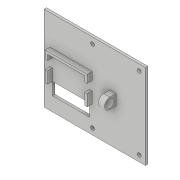
# Autodesk Inventor part: middleBase
Saved by Autodesk Inventor 2019 (Build 230136000, 136)
## iProperties
Created: 2021-03-03
Part Number: middleBase
Material: Generic
Document SubType Name: Modeling
Designer: LuoYi
Density: 1 g/cm^3
Appearance: Default
Author: LuoYi
Autodesk Inventor part; units mm, degrees
ref_plane "YZ Plane" through (0, 0, 0) normal (1, 0, 0) x (0, 1, 0)
sketch "Sketch1" plane through (0, 0, 0) normal (0, 0, 1) x (1, 0, 0)
  line L0 (0, 0) -> (83.5, 0)
  line L1 (83.5, 0) -> (83.5, 70)
  line L2 (83.5, 70) -> (0, 70)
  line L3 (0, 70) -> (0, 0)
  dimension "d0" = 70
  dimension "d1" = 83.5
  constraints: 8 end point, 2 parallel, 1 horizontal, 1 perpendicular
  measures "d0" distance of L2.end L0.start
  measures "d1" distance of L0.start L0.end
extrude "Extrusion1" add sketch "Sketch1" along normal blind 2
sketch "Sketch2" plane through (0, 0, 2) normal (0, 0, 1) x (1, 0, 0)
  line L0 (0, 70) -> (0, 0) projected
  line L1 (0, 35) -> (83.5, 35) construction
  line L2 (83.5, 0) -> (83.5, 70) projected
  line L3 (6.95, 31.4) -> (-5, 31.4) construction
  line L4 (-5, 31.4) -> (-5, 38.6) construction
  line L5 (-5, 38.6) -> (6.95, 38.6) construction
  line L6 (6.95, 38.6) -> (6.95, 31.4) construction
  line L7 (6.95, 31.4) -> (-5, 38.6) construction
  line L8 (-5, 31.4) -> (6.95, 38.6) construction
  line L9 (49.5, 34.65) -> (49.5, 29.45) construction
  line L10 (6.95, 31.4) -> (4.95, 31.4)
  line L11 (4.95, 31.4) -> (4.95, 21.85)
  line L12 (4.95, 21.85) -> (6.95, 21.85)
  line L13 (6.95, 21.85) -> (6.95, 31.4)
  line L14 (6.95, 38.6) -> (4.95, 38.6)
  line L15 (4.95, 38.6) -> (4.95, 45.2)
  line L16 (4.95, 45.2) -> (6.95, 45.2)
  line L17 (6.95, 45.2) -> (6.95, 38.6)
  line L18 (6.95, 45.2) -> (37.55, 45.2)
  line L19 (37.55, 45.2) -> (37.55, 43.2)
  line L20 (37.55, 43.2) -> (6.95, 43.2)
  line L21 (6.95, 43.2) -> (6.95, 45.2)
  line L22 (37.55, 45.2) -> (39.55, 45.2)
  line L23 (39.55, 45.2) -> (39.55, 38.6)
  line L24 (39.55, 38.6) -> (37.55, 38.6)
  line L25 (37.55, 38.6) -> (37.55, 45.2)
  line L26 (37.55, 31.4) -> (39.55, 31.4)
  line L27 (39.55, 31.4) -> (39.55, 21.85)
  line L28 (39.55, 21.85) -> (37.55, 21.85)
  line L29 (37.55, 21.85) -> (37.55, 31.4)
  line L30 (6.95, 21.85) -> (37.55, 21.85)
  line L31 (37.55, 21.85) -> (37.55, 11.6)
  line L32 (37.55, 11.6) -> (6.95, 11.6)
  line L33 (6.95, 11.6) -> (6.95, 21.85)
  point P0 (0.975, 35)
  dimension "d8" = 7.2
  dimension "d13" = 11.95
  dimension "d14" = 5
  dimension "d19" = 2
  dimension "d20" = 23.4
  dimension "d21" = 10.25
  dimension "d22" = 30.6
  dimension "d23" = 2
  dimension "d24" = 2
  dimension "d25" = 33.6
  dimension "d30" = 11.95
  constraints: 64 end point, 14 parallel, 8 point on line, 7 horizontal, 7 perpendicular, 4 midpoint
  measures "d8" distance between parallel lines of L3 L5
  measures "d13" distance between parallel lines of L6 L4
  measures "d14" distance between parallel lines of L0 L4
  measures "d19" distance between parallel lines of L15 L17
  measures "d20" distance between parallel lines of L32 L1
  measures "d21" distance between parallel lines of L32 L30
  measures "d22" distance between parallel lines of L25 L17
  measures "d23" distance between parallel lines of L25 L23
  measures "d24" distance between parallel lines of L20 L18
  measures "d25" distance between parallel lines of L32 L18
  measures "d30" distance between parallel lines of L25 L9
extrude "Extrusion2" add sketch "Sketch2" along normal blind 4 contours L13 L12 L11 L10 | L29 L26 L27 L28 | L14 L15 L16 L17 | L17 L18 L19 L20 | L19 L22 L23 L24 L25
extrude "Extrusion3" cut sketch "Sketch2" against normal blind 2 contours L30 L31 L32 L33
ref_plane "Work Plane1" through (54.5, 0, 0) normal (-1, 0, 0) x (0, 0, 1)
sketch "Sketch3" plane through (54.5, 0, 0) normal (-1, 0, 0) x (0, 0, 1)
  arc A0 (7.25, 30.5) -> (7.25, 39.5) centre (7.25, 35) ccw
  circle A1 centre (7.25, 35) radius 3.5
  line L0 (2, 21.85) -> (2, 31.4) projected
  line L1 (7.25, 39.5) -> (2, 39.5)
  line L2 (2, 39.5) -> (2, 30.5)
  line L3 (2, 30.5) -> (7.25, 30.5)
  line L4 (7.25, 30.5) -> (7.25, 39.5) construction
  arc A2 (7.25, 39.5) -> (7.25, 30.5) centre (7.25, 35) ccw construction
  line L5 (2, 38.6) -> (6, 38.6) projected
  line L6 (2, 31.4) -> (6, 31.4) projected
  line L7 (6, 38.6) -> (6, 31.4) construction
  line L8 (6, 35) -> (7.25, 35) construction
  point P0 (0, 0)
  dimension "d32" = 9
  dimension "d33" = 7
  dimension "d34" = 5.25
  constraints: 12 end point, 4 point on circle, 3 centre point, 2 horizontal, 2 parallel, 1 coincident, 1 midpoint, 1 perpendicular, 1 point on line, 1 tangent, 1 vertical
  measures "d32" distance between parallel lines of L3 L1
  measures "d33" diameter of A1
  measures "d34" distance between parallel lines of L2 L4
ref_plane "Work Plane2" through (0, 0, 7.25) normal (0, 0, 1) x (1, 0, 0)
sketch "Sketch4" plane through (0, 0, 7.25) normal (0, 0, 1) x (1, 0, 0)
  line L0 (39.55, 38.6) -> (37.55, 38.6) projected
  line L1 (37.55, 31.4) -> (39.55, 31.4) projected
  line L2 (39.55, 38.6) -> (39.55, 31.4) construction
  line L3 (39.55, 35) -> (54.5, 35) construction
  line L4 (54.5, 35) -> (59.5, 35)
  point P0 (0, 0)
  dimension "d36" = 14.95
  dimension "d37" = 5
  constraints: 6 end point, 2 horizontal, 1 midpoint, 1 vertical
  measures "d36" distance of L3.start L3.end
  measures "d37" distance of L3.end L4.end
sweep "Sweep1" add profiles "Sketch3" path "Sketch4" path curves L4
sketch "Sketch7" plane through (0, 0, 2) normal (0, 0, 1) x (1, 0, 0)
  line L0 (40, 65) -> (78.5, 65) construction
  line L1 (78.5, 65) -> (78.5, 5) construction
  line L2 (78.5, 5) -> (40, 5) construction
  line L3 (40, 5) -> (40, 65) construction
  line L4 (83.5, 70) -> (0, 70) projected
  line L5 (0, 70) -> (0, 0) projected
  line L6 (83.5, 0) -> (83.5, 70) projected
  line L7 (0, 0) -> (83.5, 0) projected
  circle A0 centre (40, 65) radius 1.6
  circle A1 centre (78.5, 65) radius 1.6
  circle A2 centre (40, 5) radius 1.6
  circle A3 centre (78.5, 5) radius 1.6
  dimension "d54" = 5
  dimension "d55" = 40
  dimension "d56" = 5
  dimension "d57" = 5
  dimension "d58" = 3.2
  dimension "d59" = 3.2
  dimension "d60" = 3.2
  dimension "d61" = 3.2
  constraints: 8 end point, 4 centre point, 4 coincident, 2 parallel, 1 horizontal, 1 perpendicular
  measures "d54" distance between parallel lines of L4 L0
  measures "d55" distance between parallel lines of L5 L3
  measures "d56" distance between parallel lines of L6 L1
  measures "d57" distance between parallel lines of L7 L2
  measures "d58" diameter of A0
  measures "d59" diameter of A1
  measures "d60" diameter of A2
  measures "d61" diameter of A3
extrude "Extrusion6" cut sketch "Sketch7" against normal blind 5 contours A0 | A1 | A2 | A3
sketch "Sketch8" plane through (0, 0, 2) normal (0, 0, 1) x (1, 0, 0)
  circle A0 centre (40, 65) radius 1.6 projected
  line L0 (40, 68.4641) -> (43, 66.7321)
  line L1 (43, 66.7321) -> (43, 63.2679)
  line L2 (43, 63.2679) -> (40, 61.5359)
  line L3 (40, 61.5359) -> (37, 63.2679)
  line L4 (37, 63.2679) -> (37, 66.7321)
  line L5 (37, 66.7321) -> (40, 68.4641)
  line L6 (40, 69.6188) -> (44, 67.3094)
  line L7 (44, 67.3094) -> (44, 62.6906)
  line L8 (44, 62.6906) -> (40, 60.3812)
  line L9 (40, 60.3812) -> (36, 62.6906)
  line L10 (36, 62.6906) -> (36, 67.3094)
  line L11 (36, 67.3094) -> (40, 69.6188)
  circle A1 centre (78.5, 5) radius 1.6 projected
  line L12 (40, 65) -> (78.5, 65) construction
  line L13 (78.5, 65) -> (78.5, 5) construction
  line L14 (78.5, 5) -> (40, 5) construction
  line L15 (40, 5) -> (40, 65) construction
  line L16 (78.5, 61.5359) -> (75.5, 63.2679)
  line L17 (75.5, 63.2679) -> (75.5, 66.7321)
  line L18 (75.5, 66.7321) -> (78.5, 68.4641)
  line L19 (78.5, 68.4641) -> (81.5, 66.7321)
  line L20 (81.5, 66.7321) -> (81.5, 63.2679)
  line L21 (81.5, 63.2679) -> (78.5, 61.5359)
  line L22 (78.5, 60.3812) -> (74.5, 62.6906)
  line L23 (74.5, 62.6906) -> (74.5, 67.3094)
  line L24 (74.5, 67.3094) -> (78.5, 69.6188)
  line L25 (78.5, 69.6188) -> (82.5, 67.3094)
  line L26 (82.5, 67.3094) -> (82.5, 62.6906)
  line L27 (82.5, 62.6906) -> (78.5, 60.3812)
  line L28 (78.5, 8.4641) -> (81.5, 6.7321)
  line L29 (81.5, 6.7321) -> (81.5, 3.2679)
  line L30 (81.5, 3.2679) -> (78.5, 1.5359)
  line L31 (78.5, 1.5359) -> (75.5, 3.2679)
  line L32 (75.5, 3.2679) -> (75.5, 6.7321)
  line L33 (75.5, 6.7321) -> (78.5, 8.4641)
  line L34 (78.5, 9.6188) -> (82.5, 7.3094)
  line L35 (82.5, 7.3094) -> (82.5, 2.6906)
  line L36 (82.5, 2.6906) -> (78.5, 0.3812)
  line L37 (78.5, 0.3812) -> (74.5, 2.6906)
  line L38 (74.5, 2.6906) -> (74.5, 7.3094)
  line L39 (74.5, 7.3094) -> (78.5, 9.6188)
  line L40 (40, 9.6188) -> (44, 7.3094)
  line L41 (44, 7.3094) -> (44, 2.6906)
  line L42 (44, 2.6906) -> (40, 0.3812)
  line L43 (40, 0.3812) -> (36, 2.6906)
  line L44 (36, 2.6906) -> (36, 7.3094)
  line L45 (36, 7.3094) -> (40, 9.6188)
  line L46 (40, 8.4641) -> (43, 6.7321)
  line L47 (43, 6.7321) -> (43, 3.2679)
  line L48 (43, 3.2679) -> (40, 1.5359)
  line L49 (40, 1.5359) -> (37, 3.2679)
  line L50 (37, 3.2679) -> (37, 6.7321)
  line L51 (37, 6.7321) -> (40, 8.4641)
  point P0 (0, 0)
  dimension "d64" = 6
  dimension "d65" = 1
  dimension "d66" = 6
  dimension "d67" = 1
  dimension "d68" = 6
  dimension "d69" = 1
  dimension "d70" = 1
  dimension "d71" = 6
  constraints: 104 end point, 8 coincident, 7 point on line, 2 parallel, 1 horizontal, 1 perpendicular, 104 other
  measures "d64" distance between parallel lines of L4 L1
  measures "d65" distance between parallel lines of L7 L1
  measures "d66" distance between parallel lines of L50 L47
  measures "d67" distance between parallel lines of L41 L47
  measures "d68" distance between parallel lines of L29 L32
  measures "d69" distance between parallel lines of L35 L29
  measures "d70" distance between parallel lines of L26 L20
  measures "d71" distance between parallel lines of L17 L20
sketch "Sketch6" plane through (0, 70, 0) normal (0, 1, 0) x (1, 0, 0)
  line L0 (83.5, -2) -> (0, -2) projected
  line L1 (79, -2) -> (79, -7.25)
  arc A0 (70, -7.25) -> (79, -7.25) centre (74.5, -7.25) ccw
  line L2 (70, -7.25) -> (70, -2)
  circle A1 centre (74.5, -7.25) radius 3.5
  line L3 (39.55, -2) -> (39.55, -6) projected
  point P0 (0, 0)
  dimension "d48" = 7
  dimension "d49" = 4.5
  dimension "d50" = 5.25
  dimension "d51" = 34.95
  constraints: 4 end point, 2 centre point, 2 point on circle, 2 point on line, 2 tangent, 1 coincident, 1 perpendicular, 1 vertical
  measures "d48" diameter of A1
  measures "d49" radius of A0
  measures "d50" distance of L2.start L2.end
  measures "d51" distance from line of L3 A0.centre
body "Solid1"
